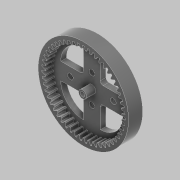
# Autodesk Inventor part: Przekładnia walcowa2
Saved by Autodesk Inventor 2021 (Build 250183000, 183)
## iProperties
CustomPartVersion: 1
Created: 2021-07-14
Part Number: Przekładnia walcowa2
Material: Tworzywo o ultrawysokiej masie cząsteczkowej, czarne
Document SubType Name: Modeling
Designer: marci
Categories: <?xml version="1.0" encoding="UTF-16"?> <MemberInstance><Categories><FamilyTemplate><FamilyTemplateParameter ValueType="xs:double" Id="1" ObjectReferenceKey="da_z" ObjectType="kUserParameterObject"/><FamilyTemplateParameter ValueType="xs:double" Id="2" ObjectReferenceKey="da_b" ObjectType="kUserParameterObject"/><FamilyTemplateParameter ValueType="xs:double" Id="3" ObjectReferenceKey="da_beta" ObjectType="kUserParameterObject"/><FamilyTemplateParameter ValueType="xs:double" Id="4" ObjectReferenceKey="da_da" ObjectType="kUserParameterObject"/><FamilyTemplateParameter ValueType="xs:double" Id="5" ObjectReferenceKey="da_aw" ObjectType="kUserParameterObject"/><FamilyTemplateParameter ValueType="xs:string" Id="6" ObjectReferenceKey="EAIAABAAAACIAQAAAAAAAIAAAAAAAAAA" ObjectType="83910656" SubObjectId="SurfaceGeometry"/></FamilyTemplate><ParamToTemplateMap><ParamToTemplate CategoryParameter="//CategoryParameter[@InternalName='046C89C9-8512-4d59-83FE-43B91F4F132A']" TemplateParameter="1"/><ParamToTemplate CategoryParameter="//CategoryParameter[@InternalName='2552DF32-E462-4b46-AEBF-C6C7768E72AC']" TemplateParameter="2"/><ParamToTemplate CategoryParameter="//CategoryParameter[@InternalName='C9EE641D-15FC-4fae-A226-E94C4372FDD7']" TemplateParameter="3"/><ParamToTemplate><ParamToTemplate CategoryParameter="//CategoryParameter[@InternalName='00B6519A-459B-49c7-AD84-2E56D39A5744']" ConstantValue="0.377035"/></ParamToTemplate><ParamToTemplate><ParamToTemplate CategoryParameter="//CategoryParameter[@InternalName='04B31F0E-C7A6-4894-AA32-9629BEFACF47']" ConstantValue="1.000000"/></ParamToTemplate><ParamToTemplate><ParamToTemplate CategoryParameter="//CategoryParameter[@InternalName='43CBEC2E-7847-49e7-A936-2F7889FCB2D9']" ConstantValue="0.250000"/></ParamToTemplate><ParamToTemplate><ParamToTemplate CategoryParameter="//CategoryParameter[@InternalName='B1EFC894-105D-4ebd-86BF-FA20ED196853']" ConstantValue="0.350000"/></ParamToTemplate><ParamToTemplate><ParamToTemplate CategoryParameter="//CategoryParameter[@InternalName='51175063-3D10-4879-93E8-6246FE8B403D']" ConstantValue="2060000000.000000"/></ParamToTemplate><ParamToTemplate><ParamToTemplate CategoryParameter="//CategoryParameter[@InternalName='A3A52E27-4454-46a9-B0BD-C932399B70AF']" ConstantValue="0.300000"/></ParamToTemplate><ParamToTemplate><ParamToTemplate CategoryParameter="//CategoryParameter[@InternalName='91B76062-C214-41d9-B1B9-14D2AB99603D']" ConstantValue="0.275000"/></ParamToTemplate><ParamToTemplate><ParamToTemplate CategoryParameter="//CategoryParameter[@InternalName='374E806E-8B8A-4dda-A9AA-1039D6500AD2']" ConstantValue="3.636364"/></ParamToTemplate><ParamToTemplate><ParamToTemplate CategoryParameter="//CategoryParameter[@InternalName='2D373A89-B862-43d6-8D0B-0CBF12AB9F6C']" ConstantValue="0.349066"/></ParamToTemplate><ParamToTemplate CategoryParameter="//CategoryParameter[@InternalName='37777632-D6A2-4fac-9D53-DB8ACD95C989']" TemplateParameter="4"/><ParamToTemplate CategoryParameter="//CategoryParameter[@InternalName='FD1017F1-B727-4f7e-9707-0F86F1FF9423']" TemplateParameter="5"/><ParamToTemplate><ParamToTemplate CategoryParameter="//CategoryParameter[@InternalName='9E1B4470-B2D3-4ff1-B813-535BB4CDF51A']" ConstantValue="3520000.000000"/></ParamToTemplate><ParamToTemplate><ParamToTemplate CategoryParameter="//CategoryParameter[@InternalName='F8452263-BFF6-458c-9FB1-07C4B99E95CD']" ConstantValue="11400000.000000"/></ParamToTemplate><ParamToTemplate><ParamToTemplate CategoryParameter="//CategoryParameter[@InternalName='3E3BB259-FD49-497f-8171-6EBC954A3479']" ConstantValue="2.000000"/></ParamToTemplate><ParamToTemplate CategoryParameter="//CategoryParameter[@InternalName='27C3BAF2-7550-4e4b-AE2C-0DB134B7D9B7']" TemplateParameter="6"/></ParamToTemplateMap><Category DisplayName="Gear" InternalName="DC85795E-93AB-48d5-8EEE-5A27447B64BD" Mnemonic="Gear"><CategoryParameter DisplayName="z" InternalName="046C89C9-8512-4d59-83FE-43B91F4F132A" Mnemonic="z"/><CategoryParameter DisplayName="b" InternalName="2552DF32-E462-4b46-AEBF-C6C7768E72AC" Mnemonic="b"/><CategoryParameter DisplayName="||b|" InternalName="C9EE641D-15FC-4fae-A226-E94C4372FDD7" Mnemonic="beta"/><CategoryParameter DisplayName="x" InternalName="00B6519A-459B-49c7-AD84-2E56D39A5744" Mnemonic="x"/><CategoryParameter DisplayName="a*" InternalName="04B31F0E-C7A6-4894-AA32-9629BEFACF47" Mnemonic="a"/><CategoryParameter DisplayName="c*" InternalName="43CBEC2E-7847-49e7-A936-2F7889FCB2D9" Mnemonic="c"/><CategoryParameter DisplayName="r|.f|*" InternalName="B1EFC894-105D-4ebd-86BF-FA20ED196853" Mnemonic="rf"/><CategoryParameter DisplayName="E" InternalName="51175063-3D10-4879-93E8-6246FE8B403D" Mnemonic="E"/><CategoryParameter DisplayName="||m|" InternalName="A3A52E27-4454-46a9-B0BD-C932399B70AF" Mnemonic="mi"/><Category DisplayName="SpurGear" InternalName="26C5A22E-A91E-4dfd-A3B3-23CCAFAE1764" Mnemonic="SpurGear"><CategoryParameter DisplayName="m" InternalName="91B76062-C214-41d9-B1B9-14D2AB99603D" Mnemonic="m"/><CategoryParameter DisplayName="P" InternalName="374E806E-8B8A-4dda-A9AA-1039D6500AD2" Mnemonic="PP"/><CategoryParameter DisplayName="||a|" InternalName="2D373A89-B862-43d6-8D0B-0CBF12AB9F6C" Mnemonic="alpha"/><CategoryParameter DisplayName="d|.a|" InternalName="37777632-D6A2-4fac-9D53-DB8ACD95C989" Mnemonic="da"/><CategoryParameter DisplayName="a|.w|" InternalName="FD1017F1-B727-4f7e-9707-0F86F1FF9423" Mnemonic="aw"/><CategoryParameter DisplayName="||s||.Flim|" InternalName="9E1B4470-B2D3-4ff1-B813-535BB4CDF51A" Mnemonic="sFlim"/><CategoryParameter DisplayName="||s||.Hlim|" InternalName="F8452263-BFF6-458c-9FB1-07C4B99E95CD" Mnemonic="sHlim"/><CategoryParameter DisplayName="typ" InternalName="3E3BB259-FD49-497f-8171-6EBC954A3479" Mnemonic="type"/><CategoryParameter DisplayName="PitchDiameter" InternalName="27C3BAF2-7550-4e4b-AE2C-0DB134B7D9B7" Mnemonic="IDS_PITCHDIAM"/></Category></Category></Categories></MemberInstance>
Density: 0.94 g/cm^3
Appearance: Gładki — czarny
Mass: 201.658 g
Surface Area: 638.402 cm^2
Volume: 214.529 cm^3
Author: marci
Autodesk Inventor part; units mm, degrees
ref_plane "Work Plane2" through (0, 0, 10) normal (0, 0, 1) x (1, 0, 0)
ref_plane "Płaszczyzna konstrukcyjna12" through (0, 0, 0) normal (0, 0, -1) x (-1, 0, 0)
ref_plane "Work Plane8" through (0, 0, 0) normal (0.9981, 0.0616, 0) x (0, 0, 1)
ref_plane "Work Plane9" through (0, 0, 0) normal (1, 0, 0) x (0, 1, 0)
ref_plane "Płaszczyzna konstrukcyjna11" through (0, 0, 0) normal (0, 0, -1) x (-1, 0, 0)
ref_plane "Płaszczyzna konstrukcyjna13" through (0, 0, 20) normal (0, 0, 1) x (1, 0, 0)
sketch "Szkic4" plane through (0, 0, 20) normal (0, 0, 1) x (1, 0, 0)
  circle A0 centre (0, 0) radius 80 projected
  arc A1 (-10.2063, 73.1666) -> (-11.4177, 66.755) centre (21.1633, 63.9195) ccw projected
  arc A2 (-11.4177, 66.755) -> (-13.468, 66.3717) centre (0, 0) ccw projected
  arc A3 (-13.468, 66.3717) -> (-16.9137, 71.9127) centre (-42.8246, 51.9581) ccw projected
  arc A4 (-16.9137, 71.9127) -> (-19.1203, 71.3578) centre (0, 0) ccw projected
  arc A5 (-19.1203, 71.3578) -> (-19.5345, 64.8459) centre (13.1479, 66.0357) ccw projected
  arc A6 (-19.5345, 64.8459) -> (-21.5222, 64.2136) centre (0, 0) ccw projected
  arc A7 (-21.5222, 64.2136) -> (-25.6228, 69.2892) centre (-48.885, 46.3016) ccw projected
  arc A8 (-25.6228, 69.2892) -> (-27.7444, 68.4673) centre (0, 0) ccw projected
  arc A9 (-27.7444, 68.4673) -> (-27.3553, 61.9538) centre (4.9333, 67.1509) ccw projected
  arc A10 (-27.3553, 61.9538) -> (-29.2502, 61.082) centre (0, 0) ccw projected
  arc A11 (-29.2502, 61.082) -> (-33.9434, 65.6153) centre (-54.2044, 39.9433) ccw projected
  arc A12 (-33.9434, 65.6153) -> (-35.9479, 64.5389) centre (0, 0) ccw projected
  arc A13 (-35.9479, 64.5389) -> (-34.7613, 58.1226) centre (-3.3562, 67.2482) ccw projected
  arc A14 (-34.7613, 58.1226) -> (-36.5347, 57.0245) centre (0, 0) ccw projected
  arc A15 (-36.5347, 57.0245) -> (-41.7495, 60.9467) centre (-58.7021, 32.9794) ccw projected
  arc A16 (-41.7495, 60.9467) -> (-43.6065, 59.6321) centre (0, 0) ccw projected
  arc A17 (-43.6065, 59.6321) -> (-41.6405, 53.4103) centre (-11.5948, 66.3261) ccw projected
  arc A18 (-41.6405, 53.4103) -> (-43.2655, 52.1026) centre (0, 0) ccw projected
  arc A19 (-43.2655, 52.1026) -> (-48.9226, 55.3542) centre (-62.31, 25.5157) ccw projected
  arc A20 (-48.9226, 55.3542) -> (-50.6041, 53.8214) centre (0, 0) ccw projected
  arc A21 (-50.6041, 53.8214) -> (-47.8883, 47.8883) centre (-19.6576, 64.3985) ccw projected
  arc A22 (-47.8883, 47.8883) -> (-49.3404, 46.3909) centre (0, 0) ccw projected
  arc A23 (-49.3404, 46.3909) -> (-55.3542, 48.9226) centre (-64.9733, 17.6651) ccw projected
  arc A24 (-55.3542, 48.9226) -> (-56.8345, 47.1948) centre (0, 0) ccw projected
  arc A25 (-56.8345, 47.1948) -> (-53.4103, 41.6405) centre (-27.4224, 61.4947) ccw projected
  arc A26 (-53.4103, 41.6405) -> (-54.6673, 39.9759) centre (0, 0) ccw projected
  arc A27 (-54.6673, 39.9759) -> (-60.9467, 41.7495) centre (-66.6517, 9.5468) ccw projected
  arc A28 (-60.9467, 41.7495) -> (-62.2035, 39.8528) centre (0, 0) ccw projected
  arc A29 (-62.2035, 39.8528) -> (-58.1226, 34.7613) centre (-34.7715, 57.6587) ccw projected
  arc A30 (-58.1226, 34.7613) -> (-59.1655, 32.955) centre (0, 0) ccw projected
  arc A31 (-59.1655, 32.955) -> (-65.6153, 33.9434) centre (-67.3197, 1.2837) ccw projected
  arc A32 (-65.6153, 33.9434) -> (-66.6294, 31.9067) centre (0, 0) ccw projected
  arc A33 (-66.6294, 31.9067) -> (-61.9538, 27.3553) centre (-41.5936, 52.9487) ccw projected
  arc A34 (-61.9538, 27.3553) -> (-62.7668, 25.4344) centre (0, 0) ccw projected
  arc A35 (-62.7668, 25.4344) -> (-69.2892, 25.6228) centre (-66.9672, -6.9988) ccw projected
  arc A36 (-69.2892, 25.6228) -> (-70.0454, 23.4768) centre (0, 0) ccw projected
  arc A37 (-70.0454, 23.4768) -> (-64.8459, 19.5345) centre (-47.7851, 47.436) ccw projected
  arc A38 (-64.8459, 19.5345) -> (-65.4167, 17.5284) centre (0, 0) ccw projected
  arc A39 (-65.4167, 17.5284) -> (-71.9127, 16.9137) centre (-65.5995, -15.1753) ccw projected
  arc A40 (-71.9127, 16.9137) -> (-72.3995, 14.6911) centre (0, 0) ccw projected
  arc A41 (-72.3995, 14.6911) -> (-66.755, 11.4177) centre (-53.2522, 41.2042) ccw projected
  arc A42 (-66.755, 11.4177) -> (-67.0749, 9.3565) centre (0, 0) ccw projected
  arc A43 (-67.0749, 9.3565) -> (-73.4462, 7.9483) centre (-63.2374, -23.1217) ccw projected
  arc A44 (-73.4462, 7.9483) -> (-73.6561, 5.6827) centre (0, 0) ccw projected
  arc A45 (-73.6561, 5.6827) -> (-67.6521, 3.1277) centre (-57.9121, 34.3478) ccw projected
  arc A46 (-67.6521, 3.1277) -> (-67.7163, 1.0429) centre (0, 0) ccw projected
  arc A47 (-67.7163, 1.0429) -> (-73.8662, -1.1376) centre (-59.9167, -30.7176) ccw projected
  arc A48 (-73.8662, -1.1376) -> (-73.7962, -3.4118) centre (0, 0) ccw projected
  arc A49 (-73.7962, -3.4118) -> (-67.5237, -5.2096) centre (-61.6941, 26.9708) ccw projected
  arc A50 (-67.5237, -5.2096) -> (-67.3312, -7.2865) centre (0, 0) ccw projected
  arc A51 (-67.3312, -7.2865) -> (-73.1666, -10.2063) centre (-55.6878, -37.8478) ccw projected
  arc A52 (-73.1666, -10.2063) -> (-72.8176, -12.4546) centre (0, 0) ccw projected
  arc A53 (-72.8176, -12.4546) -> (-66.3717, -13.468) centre (-64.5409, 19.1849) ccw projected
  arc A54 (-66.3717, -13.468) -> (-65.9255, -15.5055) centre (0, 0) ccw projected
  arc A55 (-65.9255, -15.5055) -> (-71.3578, -19.1203) centre (-50.6146, -44.4043) ccw projected
  arc A56 (-71.3578, -19.1203) -> (-70.7351, -21.3087) centre (0, 0) ccw projected
  arc A57 (-70.7351, -21.3087) -> (-64.2136, -21.5222) centre (-66.4093, 11.1081) ccw projected
  arc A58 (-64.2136, -21.5222) -> (-63.5203, -23.4895) centre (0, 0) ccw projected
  arc A59 (-63.5203, -23.4895) -> (-68.4673, -27.7444) centre (-44.7742, -50.2877) ccw projected
  arc A60 (-68.4673, -27.7444) -> (-67.5804, -29.8397) centre (0, 0) ccw projected
  arc A61 (-67.5804, -29.8397) -> (-61.082, -29.2502) centre (-67.271, 2.863) ccw projected
  arc A62 (-61.082, -29.2502) -> (-60.1523, -31.1173) centre (0, 0) ccw projected
  arc A63 (-60.1523, -31.1173) -> (-64.5389, -35.9479) centre (-38.2551, -55.4088) ccw projected
  arc A64 (-64.5389, -35.9479) -> (-63.4012, -37.9183) centre (0, 0) ccw projected
  arc A65 (-63.4012, -37.9183) -> (-57.0245, -36.5347) centre (-67.113, -5.4255) ccw projected
  arc A66 (-57.0245, -36.5347) -> (-55.8724, -38.2735) centre (0, 0) ccw projected
  arc A67 (-55.8724, -38.2735) -> (-59.6321, -43.6065) centre (-31.1561, -59.6899) ccw projected
  arc A68 (-59.6321, -43.6065) -> (-58.261, -45.4222) centre (0, 0) ccw projected
  arc A69 (-58.261, -45.4222) -> (-52.1026, -43.2655) centre (-65.9375, -13.6318) ccw projected
  arc A70 (-52.1026, -43.2655) -> (-50.7456, -44.8495) centre (0, 0) ccw projected
  arc A71 (-50.7456, -44.8495) -> (-53.8214, -50.6041) centre (-23.5847, -63.0662) ccw projected
  arc A72 (-53.8214, -50.6041) -> (-52.2375, -52.2375) centre (0, 0) ccw projected
  arc A73 (-52.2375, -52.2375) -> (-46.3909, -49.3404) centre (-63.7626, -21.6314) ccw projected
  arc A74 (-46.3909, -49.3404) -> (-44.8495, -50.7456) centre (0, 0) ccw projected
  arc A75 (-44.8495, -50.7456) -> (-47.1948, -56.8345) centre (-15.6559, -65.4865) ccw projected
  arc A76 (-47.1948, -56.8345) -> (-45.4222, -58.261) centre (0, 0) ccw projected
  arc A77 (-45.4222, -58.261) -> (-39.9759, -54.6673) centre (-60.621, -29.3031) ccw projected
  arc A78 (-39.9759, -54.6673) -> (-38.2735, -55.8724) centre (0, 0) ccw projected
  arc A79 (-38.2735, -55.8724) -> (-39.8528, -62.2035) centre (-7.4897, -66.914) ccw projected
  arc A80 (-39.8528, -62.2035) -> (-37.9183, -63.4012) centre (0, 0) ccw projected
  arc A81 (-37.9183, -63.4012) -> (-32.955, -59.1655) centre (-56.5606, -36.5306) ccw projected
  arc A82 (-32.955, -59.1655) -> (-31.1173, -60.1523) centre (0, 0) ccw projected
  arc A83 (-31.1173, -60.1523) -> (-31.9067, -66.6294) centre (0.79, -67.3273) ccw projected
  arc A84 (-31.9067, -66.6294) -> (-29.8397, -67.5804) centre (0, 0) ccw projected
  arc A85 (-29.8397, -67.5804) -> (-25.4344, -62.7668) centre (-51.6427, -43.2044) ccw projected
  arc A86 (-25.4344, -62.7668) -> (-23.4895, -63.5203) centre (0, 0) ccw projected
  arc A87 (-23.4895, -63.5203) -> (-23.4768, -70.0454) centre (9.0578, -66.7199) ccw projected
  arc A88 (-23.4768, -70.0454) -> (-21.3087, -70.7351) centre (0, 0) ccw projected
  arc A89 (-21.3087, -70.7351) -> (-17.5284, -65.4167) centre (-45.9419, -49.2232) ccw projected
  arc A90 (-17.5284, -65.4167) -> (-15.5055, -65.9255) centre (0, 0) ccw projected
  arc A91 (-15.5055, -65.9255) -> (-14.6911, -72.3995) centre (17.1882, -65.1011) ccw projected
  arc A92 (-14.6911, -72.3995) -> (-12.4546, -72.8176) centre (0, 0) ccw projected
  arc A93 (-12.4546, -72.8176) -> (-9.3565, -67.0749) centre (-39.5448, -54.4958) ccw projected
  arc A94 (-9.3565, -67.0749) -> (-7.2865, -67.3312) centre (0, 0) ccw projected
  arc A95 (-7.2865, -67.3312) -> (-5.6827, -73.6561) centre (25.0581, -62.4954) ccw projected
  arc A96 (-5.6827, -73.6561) -> (-3.4118, -73.7962) centre (0, 0) ccw projected
  arc A97 (-3.4118, -73.7962) -> (-1.0429, -67.7163) centre (-32.5481, -58.9424) ccw projected
  arc A98 (-1.0429, -67.7163) -> (1.0429, -67.7163) centre (0, 0) ccw projected
  arc A99 (1.0429, -67.7163) -> (3.4118, -73.7962) centre (32.5481, -58.9424) ccw projected
  arc A100 (3.4118, -73.7962) -> (5.6827, -73.6561) centre (0, 0) ccw projected
  arc A101 (5.6827, -73.6561) -> (7.2865, -67.3312) centre (-25.0581, -62.4954) ccw projected
  arc A102 (7.2865, -67.3312) -> (9.3565, -67.0749) centre (0, 0) ccw projected
  arc A103 (9.3565, -67.0749) -> (12.4546, -72.8176) centre (39.5448, -54.4958) ccw projected
  arc A104 (12.4546, -72.8176) -> (14.6911, -72.3995) centre (0, 0) ccw projected
  arc A105 (14.6911, -72.3995) -> (15.5055, -65.9255) centre (-17.1882, -65.1011) ccw projected
  arc A106 (15.5055, -65.9255) -> (17.5284, -65.4167) centre (0, 0) ccw projected
  arc A107 (17.5284, -65.4167) -> (21.3087, -70.7351) centre (45.9419, -49.2232) ccw projected
  arc A108 (21.3087, -70.7351) -> (23.4768, -70.0454) centre (0, 0) ccw projected
  arc A109 (23.4768, -70.0454) -> (23.4895, -63.5203) centre (-9.0578, -66.7199) ccw projected
  arc A110 (23.4895, -63.5203) -> (25.4344, -62.7668) centre (0, 0) ccw projected
  arc A111 (25.4344, -62.7668) -> (29.8397, -67.5804) centre (51.6427, -43.2044) ccw projected
  arc A112 (29.8397, -67.5804) -> (31.9067, -66.6294) centre (0, 0) ccw projected
  arc A113 (31.9067, -66.6294) -> (31.1173, -60.1523) centre (-0.79, -67.3273) ccw projected
  arc A114 (31.1173, -60.1523) -> (32.955, -59.1655) centre (0, 0) ccw projected
  arc A115 (32.955, -59.1655) -> (37.9183, -63.4012) centre (56.5606, -36.5306) ccw projected
  arc A116 (37.9183, -63.4012) -> (39.8528, -62.2035) centre (0, 0) ccw projected
  arc A117 (39.8528, -62.2035) -> (38.2735, -55.8724) centre (7.4897, -66.914) ccw projected
  arc A118 (38.2735, -55.8724) -> (39.9759, -54.6673) centre (0, 0) ccw projected
  arc A119 (39.9759, -54.6673) -> (45.4222, -58.261) centre (60.621, -29.3031) ccw projected
  arc A120 (45.4222, -58.261) -> (47.1948, -56.8345) centre (0, 0) ccw projected
  arc A121 (47.1948, -56.8345) -> (44.8495, -50.7456) centre (15.6559, -65.4865) ccw projected
  arc A122 (44.8495, -50.7456) -> (46.3909, -49.3404) centre (0, 0) ccw projected
  arc A123 (46.3909, -49.3404) -> (52.2375, -52.2375) centre (63.7626, -21.6314) ccw projected
  arc A124 (52.2375, -52.2375) -> (53.8214, -50.6041) centre (0, 0) ccw projected
  arc A125 (53.8214, -50.6041) -> (50.7456, -44.8495) centre (23.5847, -63.0662) ccw projected
  arc A126 (50.7456, -44.8495) -> (52.1026, -43.2655) centre (0, 0) ccw projected
  arc A127 (52.1026, -43.2655) -> (58.261, -45.4222) centre (65.9375, -13.6318) ccw projected
  arc A128 (58.261, -45.4222) -> (59.6321, -43.6065) centre (0, 0) ccw projected
  arc A129 (59.6321, -43.6065) -> (55.8724, -38.2735) centre (31.1561, -59.6899) ccw projected
  arc A130 (55.8724, -38.2735) -> (57.0245, -36.5347) centre (0, 0) ccw projected
  arc A131 (57.0245, -36.5347) -> (63.4012, -37.9183) centre (67.113, -5.4255) ccw projected
  arc A132 (63.4012, -37.9183) -> (64.5389, -35.9479) centre (0, 0) ccw projected
  arc A133 (64.5389, -35.9479) -> (60.1523, -31.1173) centre (38.2551, -55.4088) ccw projected
  arc A134 (60.1523, -31.1173) -> (61.082, -29.2502) centre (0, 0) ccw projected
  arc A135 (61.082, -29.2502) -> (67.5804, -29.8397) centre (67.271, 2.863) ccw projected
  arc A136 (67.5804, -29.8397) -> (68.4673, -27.7444) centre (0, 0) ccw projected
  arc A137 (68.4673, -27.7444) -> (63.5203, -23.4895) centre (44.7742, -50.2877) ccw projected
  arc A138 (63.5203, -23.4895) -> (64.2136, -21.5222) centre (0, 0) ccw projected
  arc A139 (64.2136, -21.5222) -> (70.7351, -21.3087) centre (66.4093, 11.1081) ccw projected
  arc A140 (70.7351, -21.3087) -> (71.3578, -19.1203) centre (0, 0) ccw projected
  arc A141 (71.3578, -19.1203) -> (65.9255, -15.5055) centre (50.6146, -44.4043) ccw projected
  arc A142 (65.9255, -15.5055) -> (66.3717, -13.468) centre (0, 0) ccw projected
  arc A143 (66.3717, -13.468) -> (72.8176, -12.4546) centre (64.5409, 19.1849) ccw projected
  arc A144 (72.8176, -12.4546) -> (73.1666, -10.2063) centre (0, 0) ccw projected
  arc A145 (73.1666, -10.2063) -> (67.3312, -7.2865) centre (55.6878, -37.8478) ccw projected
  arc A146 (67.3312, -7.2865) -> (67.5237, -5.2096) centre (0, 0) ccw projected
  arc A147 (67.5237, -5.2096) -> (73.7962, -3.4118) centre (61.6941, 26.9708) ccw projected
  arc A148 (73.7962, -3.4118) -> (73.8662, -1.1376) centre (0, 0) ccw projected
  arc A149 (73.8662, -1.1376) -> (67.7163, 1.0429) centre (59.9167, -30.7176) ccw projected
  arc A150 (67.7163, 1.0429) -> (67.6521, 3.1277) centre (0, 0) ccw projected
  arc A151 (67.6521, 3.1277) -> (73.6561, 5.6827) centre (57.9121, 34.3478) ccw projected
  arc A152 (73.6561, 5.6827) -> (73.4462, 7.9483) centre (0, 0) ccw projected
  arc A153 (73.4462, 7.9483) -> (67.0749, 9.3565) centre (63.2374, -23.1217) ccw projected
  arc A154 (67.0749, 9.3565) -> (66.755, 11.4177) centre (0, 0) ccw projected
  arc A155 (66.755, 11.4177) -> (72.3995, 14.6911) centre (53.2522, 41.2042) ccw projected
  arc A156 (72.3995, 14.6911) -> (71.9127, 16.9137) centre (0, 0) ccw projected
  arc A157 (71.9127, 16.9137) -> (65.4167, 17.5284) centre (65.5995, -15.1753) ccw projected
  arc A158 (65.4167, 17.5284) -> (64.8459, 19.5345) centre (0, 0) ccw projected
  arc A159 (64.8459, 19.5345) -> (70.0454, 23.4768) centre (47.7851, 47.436) ccw projected
  arc A160 (70.0454, 23.4768) -> (69.2892, 25.6228) centre (0, 0) ccw projected
  arc A161 (69.2892, 25.6228) -> (62.7668, 25.4344) centre (66.9672, -6.9988) ccw projected
  arc A162 (62.7668, 25.4344) -> (61.9538, 27.3553) centre (0, 0) ccw projected
  arc A163 (61.9538, 27.3553) -> (66.6294, 31.9067) centre (41.5936, 52.9487) ccw projected
  arc A164 (66.6294, 31.9067) -> (65.6153, 33.9434) centre (0, 0) ccw projected
  arc A165 (65.6153, 33.9434) -> (59.1655, 32.955) centre (67.3197, 1.2837) ccw projected
  arc A166 (59.1655, 32.955) -> (58.1226, 34.7613) centre (0, 0) ccw projected
  arc A167 (58.1226, 34.7613) -> (62.2035, 39.8528) centre (34.7715, 57.6587) ccw projected
  arc A168 (62.2035, 39.8528) -> (60.9467, 41.7495) centre (0, 0) ccw projected
  arc A169 (60.9467, 41.7495) -> (54.6673, 39.9759) centre (66.6517, 9.5468) ccw projected
  arc A170 (54.6673, 39.9759) -> (53.4103, 41.6405) centre (0, 0) ccw projected
  arc A171 (53.4103, 41.6405) -> (56.8345, 47.1948) centre (27.4224, 61.4947) ccw projected
  arc A172 (56.8345, 47.1948) -> (55.3542, 48.9226) centre (0, 0) ccw projected
  arc A173 (55.3542, 48.9226) -> (49.3404, 46.3909) centre (64.9733, 17.6651) ccw projected
  arc A174 (49.3404, 46.3909) -> (47.8883, 47.8883) centre (0, 0) ccw projected
  arc A175 (47.8883, 47.8883) -> (50.6041, 53.8214) centre (19.6576, 64.3985) ccw projected
  arc A176 (50.6041, 53.8214) -> (48.9226, 55.3542) centre (0, 0) ccw projected
  arc A177 (48.9226, 55.3542) -> (43.2655, 52.1026) centre (62.31, 25.5157) ccw projected
  arc A178 (43.2655, 52.1026) -> (41.6405, 53.4103) centre (0, 0) ccw projected
  arc A179 (41.6405, 53.4103) -> (43.6065, 59.6321) centre (11.5948, 66.3261) ccw projected
  arc A180 (43.6065, 59.6321) -> (41.7495, 60.9467) centre (0, 0) ccw projected
  arc A181 (41.7495, 60.9467) -> (36.5347, 57.0245) centre (58.7021, 32.9794) ccw projected
  arc A182 (36.5347, 57.0245) -> (34.7613, 58.1226) centre (0, 0) ccw projected
  arc A183 (34.7613, 58.1226) -> (35.9479, 64.5389) centre (3.3562, 67.2482) ccw projected
  arc A184 (35.9479, 64.5389) -> (33.9434, 65.6153) centre (0, 0) ccw projected
  arc A185 (33.9434, 65.6153) -> (29.2502, 61.082) centre (54.2044, 39.9433) ccw projected
  arc A186 (29.2502, 61.082) -> (27.3553, 61.9538) centre (0, 0) ccw projected
  arc A187 (27.3553, 61.9538) -> (27.7444, 68.4673) centre (-4.9333, 67.1509) ccw projected
  arc A188 (27.7444, 68.4673) -> (25.6228, 69.2892) centre (0, 0) ccw projected
  arc A189 (25.6228, 69.2892) -> (21.5222, 64.2136) centre (48.885, 46.3016) ccw projected
  arc A190 (21.5222, 64.2136) -> (19.5345, 64.8459) centre (0, 0) ccw projected
  arc A191 (19.5345, 64.8459) -> (19.1203, 71.3578) centre (-13.1479, 66.0357) ccw projected
  arc A192 (19.1203, 71.3578) -> (16.9137, 71.9127) centre (0, 0) ccw projected
  arc A193 (16.9137, 71.9127) -> (13.468, 66.3717) centre (42.8246, 51.9581) ccw projected
  arc A194 (13.468, 66.3717) -> (11.4177, 66.755) centre (0, 0) ccw projected
  arc A195 (11.4177, 66.755) -> (10.2063, 73.1666) centre (-21.1633, 63.9195) ccw projected
  arc A196 (10.2063, 73.1666) -> (7.9483, 73.4462) centre (0, 0) ccw projected
  arc A197 (7.9483, 73.4462) -> (5.2096, 67.5237) centre (36.1149, 56.8269) ccw projected
  arc A198 (5.2096, 67.5237) -> (3.1277, 67.6521) centre (0, 0) ccw projected
  arc A199 (3.1277, 67.6521) -> (1.1376, 73.8662) centre (-28.8578, 60.8343) ccw projected
  arc A200 (1.1376, 73.8662) -> (-1.1376, 73.8662) centre (0, 0) ccw projected
  arc A201 (-1.1376, 73.8662) -> (-3.1277, 67.6521) centre (28.8578, 60.8343) ccw projected
  arc A202 (-3.1277, 67.6521) -> (-5.2096, 67.5237) centre (0, 0) ccw projected
  arc A203 (-5.2096, 67.5237) -> (-7.9483, 73.4462) centre (-36.1149, 56.8269) ccw projected
  arc A204 (-7.9483, 73.4462) -> (-10.2063, 73.1666) centre (0, 0) ccw projected
extrude "Wyciągnięcie proste2" add sketch "Szkic4" along normal blind 15
sketch "Szkic5" plane through (0, 0, 20) normal (0, 0, -1) x (-1, 0, 0)
  circle A0 centre (0, 0) radius 80
  constraints: 1 centre point, 1 coincident
extrude "Wyciągnięcie proste3" add sketch "Szkic5" along normal blind 5
sketch "Szkic6" plane through (0, 0, 20) normal (0, 0, 1) x (1, 0, 0)
  circle A0 centre (0, 0) radius 4
  dimension "d54" = 8
  constraints: 1 centre point, 1 coincident
  measures "d54" diameter of A0
extrude "Wyciągnięcie proste4" cut sketch "Szkic6" against normal blind 10
sketch "Szkic7" plane through (0, 0, 20) normal (0, 0, 1) x (1, 0, 0)
  circle A0 centre (0, 0) radius 7
  circle A1 centre (0, 0) radius 4
  dimension "d57" = 14
  dimension "d80" = 8
  constraints: 2 centre point, 2 coincident
  measures "d57" diameter of A0
  measures "d80" diameter of A1
extrude "Wyciągnięcie proste5" add sketch "Szkic7" along normal blind 16.5
sketch "Szkic8" plane through (0, 0, 20) normal (0, 0, 1) x (1, 0, 0)
  line L0 (-20, -15) -> (-55, -15)
  circle A0 centre (0, 0) radius 5 projected
  line L1 (-15, -20) -> (-15, -55)
  arc A1 (-55, -15) -> (-15, -55) centre (-15, -15) ccw
  arc A2 (-15, -20) -> (-20, -15) centre (-20, -20) ccw
  line L2 (15, -20) -> (15, -55)
  arc A3 (15, -55) -> (55, -15) centre (15, -15) ccw
  line L3 (20, -15) -> (55, -15)
  arc A4 (20, -15) -> (15, -20) centre (20, -20) ccw
  line L4 (20, 15) -> (55, 15)
  arc A5 (55, 15) -> (15, 55) centre (15, 15) ccw
  line L5 (15, 20) -> (15, 55)
  arc A6 (15, 20) -> (20, 15) centre (20, 20) ccw
  line L6 (-15, 20) -> (-15, 55)
  arc A7 (-15, 55) -> (-55, 15) centre (-15, 15) ccw
  line L7 (-20, 15) -> (-55, 15)
  arc A8 (-20, 15) -> (-15, 20) centre (-20, 20) ccw
  point P0 (-15, -15)
  point P1 (15, -15)
  point P2 (15, 15)
  point P3 (-15, 15)
  dimension "d60" = 15
  dimension "d63" = 15
  dimension "d65" = 40
  dimension "d66" = 5
  dimension "d69" = 360
  constraints: 16 end point, 16 point on circle, 8 centre point, 8 point on line, 4 coincident, 2 tangent, 1 horizontal, 1 vertical, 45 other
  measures "d60" distance from line of point (0, 0) L0
  measures "d63" distance from line of point (0, 0) L1
  measures "d65" radius of A1
  measures "d66" radius of A2
extrude "Wyciągnięcie proste6" cut sketch "Szkic8" against normal blind 10 contours A2 L1 A1 L0 | A4 L3 A3 L2 | A6 L5 A5 L4 | A8 L7 A7 L6
sketch "Szkic9" plane through (0, 0, 15) normal (0, 0, -1) x (-1, 0, 0)
  point P0 (-30.0009, 61)
hole "Otwór1" at (30.0009, 61, 15) direction (0, 0, 1) diameter 4.917 depth 3.0366 tip angle 120 thread size "M6x1" class "6H" standard "ISO Metric profile"
sketch "Szkic10" plane through (0, 0, 15) normal (0, 0, -1) x (-1, 0, 0)
  circle A0 centre (0, 0) radius 80
  arc A1 (-15, 55) -> (-55, 15) centre (-15, 15) ccw projected
  line L0 (-20, 15) -> (-55, 15) projected
  arc A2 (-20, 15) -> (-15, 20) centre (-20, 20) ccw projected
  line L1 (-15, 55) -> (-15, 20) projected
  line L2 (15, 20) -> (15, 55) projected
  arc A3 (55, 15) -> (15, 55) centre (15, 15) ccw projected
  line L3 (55, 15) -> (20, 15) projected
  arc A4 (15, 20) -> (20, 15) centre (20, 20) ccw projected
  line L4 (20, -15) -> (55, -15) projected
  arc A5 (15, -55) -> (55, -15) centre (15, -15) ccw projected
  line L5 (15, -55) -> (15, -20) projected
  arc A6 (20, -15) -> (15, -20) centre (20, -20) ccw projected
  arc A7 (-15, -20) -> (-20, -15) centre (-20, -20) ccw projected
  line L6 (-15, -20) -> (-15, -55) projected
  line L7 (-55, -15) -> (-20, -15) projected
  arc A8 (-55, -15) -> (-15, -55) centre (-15, -15) ccw projected
  circle A9 centre (0, 0) radius 4 projected
  constraints: 1 centre point, 1 coincident
extrude "Wyciągnięcie proste7" add sketch "Szkic10" along normal blind 5
sketch "Szkic11" plane through (0, 0, 10) normal (0, 0, -1) x (-1, 0, 0)
  circle A0 centre (-38, 0) radius 3
  circle A1 centre (38, 0) radius 3
  circle A2 centre (0, 25) radius 3
  circle A3 centre (0, -25) radius 3
  circle A4 centre (0, 0) radius 4 projected
  dimension "d83" = 6
  dimension "d84" = 6
  dimension "d85" = 6
  dimension "d86" = 6
  dimension "d87" = 38
  dimension "d88" = 38
  dimension "d89" = 25
  dimension "d90" = 25
  constraints: 4 centre point
  measures "d83" diameter of A0
  measures "d84" diameter of A1
  measures "d85" diameter of A2
  measures "d86" diameter of A3
  measures "d87" distance of A4.centre A0.centre
  measures "d88" distance of A4.centre A1.centre
  measures "d89" distance of A2.centre A4.centre
  measures "d90" distance of A3.centre A4.centre
extrude "Wyciągnięcie proste8" cut sketch "Szkic11" against normal blind 10 contours A0 | A1 | A2 | A3
sketch "Szkic12" plane through (0, 0, 20) normal (0, 0, 1) x (1, 0, 0)
  circle A0 centre (0, 25) radius 3 projected
  circle A1 centre (0, 25) radius 5
  circle A2 centre (38, 0) radius 3 projected
  circle A3 centre (38, 0) radius 5
  circle A4 centre (0, -25) radius 3 projected
  circle A5 centre (0, -25) radius 5
  circle A6 centre (-38, 0) radius 3 projected
  circle A7 centre (-38, 0) radius 5
  point P0 (0, 0)
  dimension "d93" = 10
  dimension "d94" = 10
  dimension "d95" = 10
  dimension "d96" = 10
  constraints: 4 centre point, 4 coincident
  measures "d93" diameter of A1
  measures "d94" diameter of A3
  measures "d95" diameter of A5
  measures "d96" diameter of A7
extrude "Wyciągnięcie proste9" cut sketch "Szkic12" against normal blind 4.5 contours A0 | A1 | A2 | A3 | A5 | A7
body "Solid1"
